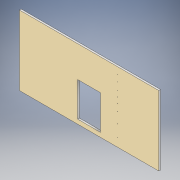
# Autodesk Inventor part: Model 2 door
Saved by Autodesk Inventor 2017 (Build 210142000, 142)
## iProperties
Created: 2017-06-12
Part Number: Model 2 door
Material: Generic
Document SubType Name: Modeling
Designer: cas7
Density: 1 g/cm^3
Appearance: Default
Author: cas7
Autodesk Inventor part; units mm, degrees
ref_plane "YZ Plane" through (0, 0, 0) normal (1, 0, 0) x (0, 1, 0)
ref_plane "XZ Plane" through (0, 0, 0) normal (0, 1, 0) x (-1, 0, 0)
ref_plane "XY Plane" through (0, 0, 0) normal (0, 0, 1) x (1, 0, 0)
sketch "Sketch3" plane through (0, 0, 0) normal (0, 0, 1) x (1, 0, 0)
  line L0 (0, 0) -> (1219.2, 0)
  line L1 (1219.2, 0) -> (1219.2, 609.6)
  line L2 (1219.2, 609.6) -> (0, 609.6)
  line L3 (0, 609.6) -> (0, 0)
  line L4 (0, 0) -> (0, 38.1)
  line L5 (509.6, 38.1) -> (709.6, 38.1)
  line L6 (609.6, 38.1) -> (509.6, 38.1)
  line L7 (509.6, 38.1) -> (509.6, 338.1)
  line L8 (509.6, 338.1) -> (709.6, 338.1)
  line L9 (709.6, 338.1) -> (709.6, 38.1)
  line L10 (609.6, 38.1) -> (709.6, 38.1)
  dimension "d7" = 1219.2
  dimension "d8" = 609.6
  dimension "d9" = 38.1
  dimension "d10" = 100
  dimension "d11" = 300
  dimension "d12" = 200
  constraints: 22 end point, 4 perpendicular, 2 parallel, 1 collinear, 1 horizontal, 1 midpoint, 1 point on line
  measures "d7" distance of L2.end L1.end
  measures "d8" distance of L1.end L0.end
  measures "d9" distance of L0.start L4.end
  measures "d10" distance of L5.start L6.start
  measures "d11" distance of L5.start L7.end
  measures "d12" distance of L7.end L8.end
extrude "Extrusion2" add sketch "Sketch3" along normal blind 15.875
sketch "Sketch4" plane through (0, 0, 15.875) normal (0, 0, 1) x (1, 0, 0)
  line L0 (0, 609.6) -> (0, 0) projected
  line L1 (0, 609.6) -> (859.6758, 609.6)
  line L2 (1219.2, 609.6) -> (0, 609.6) projected
  point P0 (859.6758, 549.275)
  point P1 (859.6758, 495.3)
  point P2 (859.6758, 431.8)
  point P3 (859.6758, 330.2)
  point P4 (859.6758, 381)
  point P5 (859.6758, 269.875)
  point P6 (859.6758, 177.8)
  point P7 (859.6758, 76.2)
  dimension "d15" = 859.6758
  constraints: 2 end point, 1 point on line
  measures "d15" distance of L0.start L1.end
hole "Hole1" at (859.6758, 549.275, 15.875) at (859.6758, 495.3, 15.875) at (859.6758, 431.8, 15.875) at (859.6758, 330.2, 15.875) at (859.6758, 381, 15.875) at (859.6758, 269.875, 15.875) at (859.6758, 177.8, 15.875) at (859.6758, 76.2, 15.875) direction (0, 0, -1) diameter 3.175 end through all
body "Solid2"
